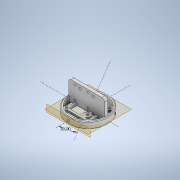
# Autodesk Inventor part: Electro_Sensor
Saved by Autodesk Inventor 2020 (Build 240168000, 168)
## iProperties
Created: 2020-09-03
Part Number: Electro_Sensor
Material: Generisch
Document SubType Name: Modeling
Designer: sp
Density: 1 g/cm^3
Appearance: Vorgabe
Author: sp
## iProperties of the stored document _3D-Druck.ipt
Created: 2020-09-03
Part Number: _3D-Druck
Material: Generisch
Document SubType Name: Modeling
Designer: sp
Density: 1 g/cm^3
Appearance: Vorgabe
Author: sp
Autodesk Inventor part; units mm, degrees
ref_plane "YZ Plane" through (0, 0, 0) normal (1, 0, 0) x (0, 1, 0)
sketch "Skizze1" plane through (0, 0, 0) normal (0, 1, 0) x (-1, 0, 0)
  circle A0 centre (0, 0) radius 30
  circle A1 centre (0, 0) radius 27
  dimension "d0" = 60
  dimension "d1" = 54
  constraints: 2 centre point, 2 coincident
  measures "d0" diameter of A0
  measures "d1" diameter of A1
extrude "Extrusion1" add sketch "Skizze1" along normal mid plane 10
ref_plane "Arbeitsebene1" through (0, 0, 0) normal (0, 1, 0) x (-1, 0, 0)
chamfer "Fase1" distance 1 angle 45 2 edges at (30, 5, 0) (30, -5, 0)
sketch "Skizze2" plane through (0, 0, 0) normal (0, 1, 0) x (-1, 0, 0)
  line L0 (0, 42.2301) -> (0, -36.7007) construction
  line L1 (32.6355, 0) -> (-32.6355, 0) construction
  line L2 (16.5, 34.419) -> (16.5, -40.3324) construction
  line L3 (-16.5, 35.4304) -> (-16.5, -34.8157) construction
  line L4 (23.5881, 16.5) -> (-32.0387, 16.5) construction
  line L5 (23.5881, -16.5) -> (-39.8541, -16.5) construction
  circle A0 centre (16.5, -16.5) radius 1.75
  circle A1 centre (16.5, 16.5) radius 1.75
  circle A2 centre (-16.5, 16.5) radius 1.75
  circle A3 centre (-16.5, -16.5) radius 1.75
  circle A4 centre (-16.5, 16.5) radius 3.6749
  circle A5 centre (-16.5, -16.5) radius 3.7161
  circle A6 centre (16.5, -16.5) radius 3.7
  circle A7 centre (16.5, 16.5) radius 3.6747
  point P0 (0, 0)
  dimension "d8" = 33
  dimension "d9" = 33
  dimension "d10" = 3.5
  dimension "d11" = 3.5
  dimension "d12" = 3.5
  dimension "d13" = 3.5
  constraints: 12 end point, 9 point on line, 8 centre point, 4 coincident, 3 horizontal, 3 vertical, 1 midpoint, 2 other
  measures "d8" distance between parallel lines of L3 L2
  measures "d9" distance between parallel lines of L4 L5
  measures "d10" diameter of A0
  measures "d11" diameter of A1
  measures "d12" diameter of A2
  measures "d13" diameter of A3
extrude "Extrusion2" add sketch "Skizze2" along normal mid plane 3
fillet "Rundung1" radius 2 16 edges at (-18.7043, 0.75, -19.4718) (-18.7043, -0.75, -19.4718) (-19.4718, 0.75, -18.7043) (-19.4718, -0.75, -18.7043) (-18.8927, 0.75, 19.289) (-18.8927, -0.75, 19.289) (-19.289, 0.75, 18.8927) (-19.289, -0.75, 18.8927) (18.8904, 0.75, 19.2913) (18.8904, -0.75, 19.2913) (19.2913, 0.75, 18.8904) (19.2913, -0.75, 18.8904) (19.551, 0.75, -18.6215) (19.551, -0.75, -18.6215) (18.6215, 0.75, -19.551) (18.6215, -0.75, -19.551)
sketch "Skizze3" plane through (0, 0, 0) normal (0, 1, 0) x (-1, 0, 0)
  circle A0 centre (-16.5, -16.5) radius 1.75 projected
  line L0 (16.5712, -18.25) -> (-16.5, -18.25)
  line L1 (-16.5, -18.25) -> (-16.5, -14.75)
  line L2 (-16.5, -14.75) -> (16.5712, -14.75)
  line L3 (16.5712, -14.75) -> (16.5712, -18.25)
  circle A1 centre (-16.5, 16.5) radius 1.75 projected
  line L4 (-18.25, 16.5) -> (-14.75, 16.5)
  line L5 (-14.75, 16.5) -> (-14.75, -16.5)
  line L6 (-14.75, -16.5) -> (-18.25, -16.5)
  line L7 (-18.25, -16.5) -> (-18.25, 16.5)
  circle A2 centre (16.5, 16.5) radius 1.75 projected
  line L8 (16.5, 14.75) -> (-16.8045, 14.75)
  line L9 (-16.8045, 14.75) -> (-16.8045, 18.2233)
  line L10 (-16.8045, 18.2233) -> (16.5, 18.2233)
  line L11 (16.5, 18.2233) -> (16.5, 14.75)
  circle A3 centre (-16.5, -16.5) radius 1.75 projected
  circle A4 centre (16.5, -16.5) radius 1.75 projected
  line L12 (18.25, -16.5) -> (14.75, -16.5)
  line L13 (14.75, -16.5) -> (14.75, 16.5)
  line L14 (14.75, 16.5) -> (18.25, 16.5)
  line L15 (18.25, 16.5) -> (18.25, -16.5)
  point P0 (0, 0)
  point P1 (14.75, -14.75)
  point P2 (-14.75, -14.75)
  point P3 (16.5, -18.25)
  point P4 (14.75, 14.75)
  point P5 (16.1955, 18.2233)
  point P6 (-16.1955, 18.2233)
  point P7 (-14.75, 14.75)
  point P8 (16.5712, -14.7514)
  point P9 (-16.8045, 14.7767)
  constraints: 32 end point, 8 parallel, 7 point on circle, 4 horizontal, 4 perpendicular, 2 other
extrude "Extrusion3" add sketch "Skizze3" against normal mid plane 3 contours L5 L2 L13 A4 L0 A0 | A0 L7 A1 L9 L8 L5 L2 | L13 L8 A2 L15 A4 L2 | L5 A1 L10 A2 L13 L8
ref_plane "Arbeitsebene2" through (0, 0, 30) normal (0, 0, 1) x (1, 0, 0)
sketch "Skizze4" plane through (0, 0, 30) normal (0, 0, 1) x (1, 0, 0)
  circle A0 centre (0, 0) radius 1.75
  dimension "d20" = 3.5
  constraints: 1 centre point, 1 coincident
  measures "d20" diameter of A0
extrude "Extrusion4" cut sketch "Skizze4" against normal blind 5
sketch "Skizze6" plane through (0, 0, 0) normal (0, 1, 0) x (-1, 0, 0)
  line L0 (0, 50.1563) -> (0, -65.6092) construction
  line L1 (-47.8971, 0) -> (73.2619, 0) construction
  line L2 (-30.0527, 52.0529) -> (47.8935, -82.954) construction
  point P0 (0, 0)
  point P1 (-14.9945, 25.9712)
  dimension "d24" = 30
  constraints: 6 end point, 4 point on line, 1 horizontal, 1 vertical
  measures "d24" angle of L2 L0
pattern_circular "Runde Anordnung2" count 3 over 360 about axis through (0, -10, 0) along (0, 1, 0) of "Extrusion4"
sketch "Skizze9" plane through (0, 0, 0) normal (0, 1, 0) x (-1, 0, 0)
  line L0 (-8, 44.1952) -> (-8, -71.3617) construction
  line L1 (46.3382, 0) -> (-50.9369, 0) construction
  circle A0 centre (-8, 9) radius 1.75
  circle A1 centre (-8, -9) radius 1.75
  circle A2 centre (-8, 9) radius 5
  circle A3 centre (-8, -9) radius 5
  line L2 (-6.25, 4.3163) -> (-9.75, 4.3163)
  line L3 (-9.75, 4.3163) -> (-9.75, -4.3163)
  line L4 (-9.75, -4.3163) -> (-6.25, -4.3163)
  line L5 (-6.25, -4.3163) -> (-6.25, 4.3163)
  line L6 (-6.25, 13.6837) -> (-9.75, 13.6837)
  line L7 (-9.75, 13.6837) -> (-9.75, 15.7789)
  line L8 (-9.75, 15.7789) -> (-6.25, 15.7789)
  line L9 (-6.25, 15.7789) -> (-6.25, 13.6837)
  line L10 (-6.25, -13.6837) -> (-9.75, -13.6837)
  line L11 (-9.75, -13.6837) -> (-9.75, -15.8841)
  line L12 (-9.75, -15.8841) -> (-6.25, -15.8841)
  line L13 (-6.25, -15.8841) -> (-6.25, -13.6837)
  point P0 (0, 0)
  dimension "d31" = 18
  dimension "d32" = 3.5
  dimension "d33" = 3.5
  dimension "d34" = 10
  dimension "d35" = 10
  dimension "d36" = 3.5
  dimension "d37" = 8
  constraints: 28 end point, 6 parallel, 6 point on line, 4 centre point, 4 horizontal, 4 point on circle, 3 perpendicular, 2 coincident, 1 symmetric about line, 1 vertical, 1 other
  measures "d31" distance of A1.centre A0.centre
  measures "d32" diameter of A1
  measures "d33" diameter of A0
  measures "d34" diameter of A2
  measures "d35" diameter of A3
  measures "d36" distance between parallel lines of L3 L5
  measures "d37" distance from line of point (0, 0) L0
extrude "Extrusion5" add sketch "Skizze9" along normal mid plane 3
sketch "Skizze10" plane through (0, -1.5, 0) normal (0, -1, 0) x (1, 0, 0)
  line L0 (42.1147, 0) -> (-38.983, 0) construction
  line L1 (27.5, 2.25) -> (-27.5, 2.25)
  line L2 (-27.5, 2.25) -> (-27.5, -2.25)
  line L3 (-27.5, -2.25) -> (27.5, -2.25)
  line L4 (27.5, -2.25) -> (27.5, 2.25)
  line L5 (0, 38.4937) -> (0, -45.0833) construction
  point P0 (0, 0)
  dimension "d40" = 4.5
  dimension "d41" = 55
  constraints: 12 end point, 2 horizontal, 2 parallel, 2 point on line, 1 perpendicular, 1 vertical, 2 other
  measures "d40" distance between parallel lines of L1 L3
  measures "d41" distance of L2.end L3.end
extrude "Extrusion6" add sketch "Skizze10" against normal blind 30
sketch "Skizze12" plane through (6.25, -1.5, -2.25) normal (0, 0, -1) x (-1, 0, 0)
  line L0 (13.75, 35.4125) -> (13.75, -8.4359) construction
  line L1 (-24.9564, 16) -> (44.4128, 16) construction
  line L2 (-21.25, 30) -> (33.75, 30) construction
  line L3 (33.75, 6.5) -> (33.75, 30) construction
  circle A0 centre (3.75, 5.6) radius 1.5
  circle A1 centre (3.75, 26.4) radius 1.5
  circle A2 centre (23.75, 26.4) radius 1.5
  circle A3 centre (23.75, 5.6) radius 1.5
  point P0 (6.25, 1.5)
  dimension "d44" = 14
  dimension "d45" = 20
  dimension "d46" = 3
  dimension "d47" = 20.8
  dimension "d48" = 20
  constraints: 4 centre point, 4 end point, 4 symmetric about line, 3 equal radius, 1 horizontal, 1 vertical
  measures "d44" distance between parallel lines of L2 L1
  measures "d45" distance between parallel lines of L3 L0
  measures "d46" diameter of A1
  measures "d47" distance of A0.centre A1.centre
  measures "d48" distance of A2.centre A1.centre
extrude "Extrusion7" cut sketch "Skizze12" against normal blind 5
sketch "Skizze13" plane through (-14.75, -1.5, 2.25) normal (0, 0, 1) x (1, 0, 0)
  line L0 (-18.4228, 25) -> (46.0376, 25) construction
  line L1 (14.75, 37.9202) -> (14.75, -3.331) construction
  circle A0 centre (4.75, 25) radius 1.75
  circle A1 centre (24.75, 25) radius 1.75
  line L2 (-12.75, 30) -> (42.25, 30) projected
  line L3 (-12.75, 6.5) -> (-12.75, 30) projected
  point P0 (14.75, 1.5)
  dimension "d51" = 3.5
  dimension "d52" = 3.5
  dimension "d53" = 20
  dimension "d54" = 5
  dimension "d55" = 27.5
  constraints: 4 end point, 2 centre point, 2 point on line, 1 horizontal, 1 symmetric about line, 1 vertical
  measures "d51" diameter of A0
  measures "d52" diameter of A1
  measures "d53" distance of A1.centre A0.centre
  measures "d54" distance between parallel lines of L2 L0
  measures "d55" distance between parallel lines of L3 L1
extrude "Extrusion8" cut sketch "Skizze13" against normal through all
fillet "Rundung2" radius 4 2 edges at (27.5, 28.5, 0) (-27.5, 28.5, 0)
fillet "Rundung3" radius 4 3 edges at (-26.9765, -1.5, -1.126) (-26.9765, -1.5, 1.126) (27, -1.5, 0)
